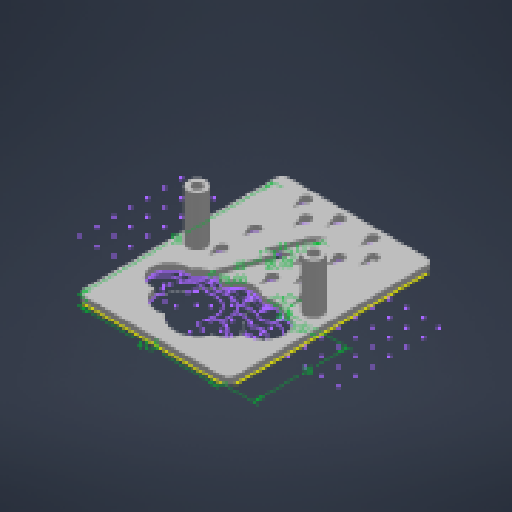
# Autodesk Inventor part: Odbiornik_top
Saved by Autodesk Inventor 2024.4 (Build 284460000, 460)
## iProperties
Created: 2026-02-27
Part Number: Odbiornik_top
Material: Ogólny
Document SubType Name: Modeling
Designer: User
Density: 1 g/cm^3
Appearance: Domyślna
Mass: 5.46546 g
Surface Area: 70.3735 cm^2
Volume: 5.46546 cm^3
Author: User
Autodesk Inventor part; units mm, degrees
ref_plane "YZ Plane" through (0, 0, 0) normal (1, 0, 0) x (0, 1, 0)
ref_plane "XZ Plane" through (0, 0, 0) normal (0, 1, 0) x (-1, 0, 0)
ref_plane "XY Plane" through (0, 0, 0) normal (0, 0, 1) x (1, 0, 0)
sketch "Szkic1" plane through (0, 0, 0) normal (0, 1, 0) x (-1, 0, 0)
  line L0 (-22.5, 30.5) -> (22.5, 30.5)
  line L1 (22.5, 30.5) -> (22.5, -30.5)
  line L2 (22.5, -30.5) -> (-22.5, -30.5)
  line L3 (-22.5, -30.5) -> (-22.5, 30.5)
  line L4 (-22.5, 30.5) -> (22.5, -30.5) construction
  line L5 (22.5, 30.5) -> (16.6, 30.5)
  line L6 (0, -30.5) -> (0, 30.5)
  line L7 (22.5, 0) -> (-22.5, 0)
  line L8 (0, 0) -> (22.5, 0)
  line L9 (22.5, 0) -> (17.38, 0)
  circle A0 centre (17.38, 0) radius 1.5
  circle A1 centre (-17.38, 0) radius 1.5
  circle A2 centre (17.38, 0) radius 2.75
  circle A3 centre (-17.38, 0) radius 2.75
  dimension "d0" = 45
  dimension "d1" = 61
  dimension "d12" = 5.12
  dimension "d13" = 3
  dimension "d14" = 30.5
  dimension "d16" = 5.5
  constraints: 20 end point, 5 midpoint, 4 centre point, 2 coincident, 2 parallel, 2 perpendicular, 2 point on line, 2 symmetric about line, 1 horizontal, 2 other
  measures "d0" distance of L1.end L2.end
  measures "d1" distance of L0.end L1.end
  measures "d12" distance of L7.start L9.end
  measures "d13" diameter of A0
  measures "d14" distance from line of L2 A0.centre
  measures "d16" diameter of A2
extrude "Wyciągnięcie proste1" add sketch "Szkic1" along normal blind 2
extrude "Wyciągnięcie proste2" add sketch "Szkic1" along normal blind 16.8 contours A3 L7 A1 | L7 A1 A3 | A2 L7 A0 | L7 A0 A2
fillet "Zaokrąglenie1" radius 2 4 edges at (-22.5, 1, -30.5) (22.5, 1, -30.5) (-22.5, 1, 30.5) (22.5, 1, 30.5)
sketch "Szkic2" plane through (0, 0, 0) normal (0, -1, 0) x (1, 0, 0)
  line L0 (-21.3296, 27.1767) -> (19.4219, 27.1767) construction
  line L1 (19.4219, 27.1767) -> (19.4219, 1.9055) construction
  line L2 (19.4219, 1.9055) -> (-21.3296, 1.9055) construction
  line L3 (-21.3296, 1.9055) -> (-21.3296, 27.1767) construction
  arc A0 (-12.0648, 18.0488) -> (-11.6976, 7.6041) centre (-12.7532, 12.7958) ccw
  arc A1 (-4.0274, 22.9506) -> (-12.0648, 18.0488) centre (-6.2944, 17.6274) ccw
  arc A2 (8.5818, 21.2572) -> (-4.0274, 22.9506) centre (1.8261, 18.7454) ccw
  arc A3 (12.8836, 16.997) -> (8.5818, 21.2572) centre (7.5717, 15.9353) ccw
  arc A4 (13.1567, 4.5998) -> (12.8836, 16.997) centre (13.0201, 10.7984) ccw
  arc A5 (5.8616, 3.9573) -> (13.1567, 4.5998) centre (8.9779, 10.3115) ccw
  arc A6 (-3.8391, 6.0403) -> (5.8616, 3.9573) centre (1.7998, 8.6711) ccw
  arc A7 (-11.6976, 7.6041) -> (-3.8391, 6.0403) centre (-7.052, 10.4219) ccw
  arc A8 (-4.2074, 7.6238) -> (1.2341, 16.8874) centre (-1.0275, 11.9859) ccw
  arc A9 (-11.7503, 10.9688) -> (-4.2074, 7.6238) centre (-7.2953, 10.8377) ccw
  arc A10 (-17.5377, 13.4696) -> (-11.6516, 9.8959) centre (-12.6699, 14.853) ccw
  arc A11 (3.697, 14.5972) -> (8.6049, 17.9558) centre (3.8701, 19.6096) ccw
  arc A12 (8.6049, 17.9558) -> (11.4505, 18.7493) centre (9.522, 20.1659) ccw
  arc A13 (4.0342, 10.11) -> (9.8976, 11.5253) centre (5.9899, 14.8611) ccw
  arc A14 (9.8976, 11.5253) -> (15.929, 15.2269) centre (12.4747, 14.0908) ccw
  arc A15 (2.5761, 7.9667) -> (9.7755, 8.6284) centre (5.7685, 12.7291) ccw
  arc A16 (9.7755, 8.6284) -> (16.9382, 14.9131) centre (13.3568, 11.7708) ccw
  arc A17 (6.5881, 21.4672) -> (5.2016, 25.1136) centre (2.4919, 21.9965) ccw
  arc A18 (8.5818, 21.2572) -> (6.5881, 21.4672) centre (7.4205, 19.8009) ccw
  arc A19 (10.5725, 13.6586) -> (9.9908, 20.782) centre (6.7774, 16.9342) ccw
  arc A20 (10.5725, 13.6586) -> (12.8792, 16.8923) centre (9.671, 16.7412) ccw
  arc A21 (15.929, 15.2269) -> (15.0518, 16.6562) centre (12.4747, 14.0908) ccw
  arc A22 (16.9382, 14.9131) -> (16.3778, 16.0107) centre (0.1209, 7.0188) ccw
  arc A23 (-11.7503, 10.9688) -> (-5.6989, 9.2808) centre (-8.2416, 11.8564) ccw
  arc A24 (-5.6989, 9.2808) -> (1.2341, 16.8874) centre (-3.3438, 14.0971) ccw
  arc A25 (-11.9834, 18.6814) -> (-11.3996, 15.8747) centre (-9.0372, 17.8302) ccw
  line L4 (-17.5377, 13.4696) -> (-17.7253, 14.625)
  circle A26 centre (12.5, 2.5) radius 1.5
  line L5 (12.5, 2.5) -> (12.5, 6.5)
  arc A27 (12.5, 6.5) -> (13.998, 2.4218) centre (38.5202, 13.7434) ccw
  arc A28 (11.002, 2.4218) -> (12.5, 6.5) centre (-13.5202, 13.7434) ccw
  line L6 (19.4219, 1.9055) -> (19.4219, -1.6866) construction
  line L7 (7.5, 2.5) -> (7.5, 6.5)
  arc A29 (7.5, 6.5) -> (8.998, 2.4218) centre (33.5202, 13.7434) ccw
  circle A30 centre (7.5, 2.5) radius 1.5
  arc A31 (6.002, 2.4218) -> (7.5, 6.5) centre (-18.5202, 13.7434) ccw
  line L8 (2.5, 2.5) -> (2.5, 6.5)
  arc A32 (2.5, 6.5) -> (3.998, 2.4218) centre (28.5202, 13.7434) ccw
  circle A33 centre (2.5, 2.5) radius 1.5
  arc A34 (1.002, 2.4218) -> (2.5, 6.5) centre (-23.5202, 13.7434) ccw
  line L9 (-2.5, 2.5) -> (-2.5, 6.5)
  arc A35 (-2.5, 6.5) -> (-1.002, 2.4218) centre (23.5202, 13.7434) ccw
  circle A36 centre (-2.5, 2.5) radius 1.5
  arc A37 (-3.998, 2.4218) -> (-2.5, 6.5) centre (-28.5202, 13.7434) ccw
  line L10 (-7.5, 2.5) -> (-7.5, 6.5)
  arc A38 (-7.5, 6.5) -> (-6.002, 2.4218) centre (18.5202, 13.7434) ccw
  circle A39 centre (-7.5, 2.5) radius 1.5
  arc A40 (-8.998, 2.4218) -> (-7.5, 6.5) centre (-33.5202, 13.7434) ccw
  line L11 (-12.5, 2.5) -> (-12.5, 6.5)
  arc A41 (-12.5, 6.5) -> (-11.002, 2.4218) centre (13.5202, 13.7434) ccw
  circle A42 centre (-12.5, 2.5) radius 1.5
  arc A43 (-13.998, 2.4218) -> (-12.5, 6.5) centre (-38.5202, 13.7434) ccw
  line L12 (12.5, -2.5) -> (12.5, 1.5)
  arc A44 (12.5, 1.5) -> (13.998, -2.5782) centre (38.5202, 8.7434) ccw
  circle A45 centre (12.5, -2.5) radius 1.5
  arc A46 (11.002, -2.5782) -> (12.5, 1.5) centre (-13.5202, 8.7434) ccw
  line L13 (7.5, -2.5) -> (7.5, 1.5)
  arc A47 (7.5, 1.5) -> (8.998, -2.5782) centre (33.5202, 8.7434) ccw
  circle A48 centre (7.5, -2.5) radius 1.5
  arc A49 (6.002, -2.5782) -> (7.5, 1.5) centre (-18.5202, 8.7434) ccw
  line L14 (2.5, -2.5) -> (2.5, 1.5)
  arc A50 (2.5, 1.5) -> (3.998, -2.5782) centre (28.5202, 8.7434) ccw
  circle A51 centre (2.5, -2.5) radius 1.5
  arc A52 (1.002, -2.5782) -> (2.5, 1.5) centre (-23.5202, 8.7434) ccw
  line L15 (-2.5, -2.5) -> (-2.5, 1.5)
  arc A53 (-2.5, 1.5) -> (-1.002, -2.5782) centre (23.5202, 8.7434) ccw
  circle A54 centre (-2.5, -2.5) radius 1.5
  arc A55 (-3.998, -2.5782) -> (-2.5, 1.5) centre (-28.5202, 8.7434) ccw
  line L16 (-7.5, -2.5) -> (-7.5, 1.5)
  arc A56 (-7.5, 1.5) -> (-6.002, -2.5782) centre (18.5202, 8.7434) ccw
  circle A57 centre (-7.5, -2.5) radius 1.5
  arc A58 (-8.998, -2.5782) -> (-7.5, 1.5) centre (-33.5202, 8.7434) ccw
  line L17 (-12.5, -2.5) -> (-12.5, 1.5)
  arc A59 (-12.5, 1.5) -> (-11.002, -2.5782) centre (13.5202, 8.7434) ccw
  circle A60 centre (-12.5, -2.5) radius 1.5
  arc A61 (-13.998, -2.5782) -> (-12.5, 1.5) centre (-38.5202, 8.7434) ccw
  line L18 (12.5, -7.5) -> (12.5, -3.5)
  arc A62 (12.5, -3.5) -> (13.998, -7.5782) centre (38.5202, 3.7434) ccw
  circle A63 centre (12.5, -7.5) radius 1.5
  arc A64 (11.002, -7.5782) -> (12.5, -3.5) centre (-13.5202, 3.7434) ccw
  line L19 (7.5, -7.5) -> (7.5, -3.5)
  arc A65 (7.5, -3.5) -> (8.998, -7.5782) centre (33.5202, 3.7434) ccw
  circle A66 centre (7.5, -7.5) radius 1.5
  arc A67 (6.002, -7.5782) -> (7.5, -3.5) centre (-18.5202, 3.7434) ccw
  line L20 (2.5, -7.5) -> (2.5, -3.5)
  arc A68 (2.5, -3.5) -> (3.998, -7.5782) centre (28.5202, 3.7434) ccw
  circle A69 centre (2.5, -7.5) radius 1.5
  arc A70 (1.002, -7.5782) -> (2.5, -3.5) centre (-23.5202, 3.7434) ccw
  line L21 (-2.5, -7.5) -> (-2.5, -3.5)
  arc A71 (-2.5, -3.5) -> (-1.002, -7.5782) centre (23.5202, 3.7434) ccw
  circle A72 centre (-2.5, -7.5) radius 1.5
  arc A73 (-3.998, -7.5782) -> (-2.5, -3.5) centre (-28.5202, 3.7434) ccw
  line L22 (-7.5, -7.5) -> (-7.5, -3.5)
  arc A74 (-7.5, -3.5) -> (-6.002, -7.5782) centre (18.5202, 3.7434) ccw
  circle A75 centre (-7.5, -7.5) radius 1.5
  arc A76 (-8.998, -7.5782) -> (-7.5, -3.5) centre (-33.5202, 3.7434) ccw
  line L23 (-12.5, -7.5) -> (-12.5, -3.5)
  arc A77 (-12.5, -3.5) -> (-11.002, -7.5782) centre (13.5202, 3.7434) ccw
  circle A78 centre (-12.5, -7.5) radius 1.5
  arc A79 (-13.998, -7.5782) -> (-12.5, -3.5) centre (-38.5202, 3.7434) ccw
  line L24 (12.5, -12.5) -> (12.5, -8.5)
  arc A80 (12.5, -8.5) -> (13.998, -12.5782) centre (38.5202, -1.2566) ccw
  circle A81 centre (12.5, -12.5) radius 1.5
  arc A82 (11.002, -12.5782) -> (12.5, -8.5) centre (-13.5202, -1.2566) ccw
  line L25 (7.5, -12.5) -> (7.5, -8.5)
  arc A83 (7.5, -8.5) -> (8.998, -12.5782) centre (33.5202, -1.2566) ccw
  circle A84 centre (7.5, -12.5) radius 1.5
  arc A85 (6.002, -12.5782) -> (7.5, -8.5) centre (-18.5202, -1.2566) ccw
  line L26 (2.5, -12.5) -> (2.5, -8.5)
  arc A86 (2.5, -8.5) -> (3.998, -12.5782) centre (28.5202, -1.2566) ccw
  circle A87 centre (2.5, -12.5) radius 1.5
  arc A88 (1.002, -12.5782) -> (2.5, -8.5) centre (-23.5202, -1.2566) ccw
  line L27 (-2.5, -12.5) -> (-2.5, -8.5)
  arc A89 (-2.5, -8.5) -> (-1.002, -12.5782) centre (23.5202, -1.2566) ccw
  circle A90 centre (-2.5, -12.5) radius 1.5
  arc A91 (-3.998, -12.5782) -> (-2.5, -8.5) centre (-28.5202, -1.2566) ccw
  line L28 (-7.5, -12.5) -> (-7.5, -8.5)
  arc A92 (-7.5, -8.5) -> (-6.002, -12.5782) centre (18.5202, -1.2566) ccw
  circle A93 centre (-7.5, -12.5) radius 1.5
  arc A94 (-8.998, -12.5782) -> (-7.5, -8.5) centre (-33.5202, -1.2566) ccw
  line L29 (-12.5, -12.5) -> (-12.5, -8.5)
  arc A95 (-12.5, -8.5) -> (-11.002, -12.5782) centre (13.5202, -1.2566) ccw
  circle A96 centre (-12.5, -12.5) radius 1.5
  arc A97 (-13.998, -12.5782) -> (-12.5, -8.5) centre (-38.5202, -1.2566) ccw
  line L30 (12.5, -17.5) -> (12.5, -13.5)
  arc A98 (12.5, -13.5) -> (13.998, -17.5782) centre (38.5202, -6.2566) ccw
  circle A99 centre (12.5, -17.5) radius 1.5
  arc A100 (11.002, -17.5782) -> (12.5, -13.5) centre (-13.5202, -6.2566) ccw
  line L31 (7.5, -17.5) -> (7.5, -13.5)
  arc A101 (7.5, -13.5) -> (8.998, -17.5782) centre (33.5202, -6.2566) ccw
  circle A102 centre (7.5, -17.5) radius 1.5
  arc A103 (6.002, -17.5782) -> (7.5, -13.5) centre (-18.5202, -6.2566) ccw
  line L32 (2.5, -17.5) -> (2.5, -13.5)
  arc A104 (2.5, -13.5) -> (3.998, -17.5782) centre (28.5202, -6.2566) ccw
  circle A105 centre (2.5, -17.5) radius 1.5
  arc A106 (1.002, -17.5782) -> (2.5, -13.5) centre (-23.5202, -6.2566) ccw
  line L33 (-2.5, -17.5) -> (-2.5, -13.5)
  arc A107 (-2.5, -13.5) -> (-1.002, -17.5782) centre (23.5202, -6.2566) ccw
  circle A108 centre (-2.5, -17.5) radius 1.5
  arc A109 (-3.998, -17.5782) -> (-2.5, -13.5) centre (-28.5202, -6.2566) ccw
  line L34 (-7.5, -17.5) -> (-7.5, -13.5)
  arc A110 (-7.5, -13.5) -> (-6.002, -17.5782) centre (18.5202, -6.2566) ccw
  circle A111 centre (-7.5, -17.5) radius 1.5
  arc A112 (-8.998, -17.5782) -> (-7.5, -13.5) centre (-33.5202, -6.2566) ccw
  line L35 (-12.5, -17.5) -> (-12.5, -13.5)
  arc A113 (-12.5, -13.5) -> (-11.002, -17.5782) centre (13.5202, -6.2566) ccw
  circle A114 centre (-12.5, -17.5) radius 1.5
  arc A115 (-13.998, -17.5782) -> (-12.5, -13.5) centre (-38.5202, -6.2566) ccw
  line L36 (12.5, -22.5) -> (12.5, -18.5)
  arc A116 (12.5, -18.5) -> (13.998, -22.5782) centre (38.5202, -11.2566) ccw
  circle A117 centre (12.5, -22.5) radius 1.5
  arc A118 (11.002, -22.5782) -> (12.5, -18.5) centre (-13.5202, -11.2566) ccw
  line L37 (7.5, -22.5) -> (7.5, -18.5)
  arc A119 (7.5, -18.5) -> (8.998, -22.5782) centre (33.5202, -11.2566) ccw
  circle A120 centre (7.5, -22.5) radius 1.5
  arc A121 (6.002, -22.5782) -> (7.5, -18.5) centre (-18.5202, -11.2566) ccw
  line L38 (2.5, -22.5) -> (2.5, -18.5)
  arc A122 (2.5, -18.5) -> (3.998, -22.5782) centre (28.5202, -11.2566) ccw
  circle A123 centre (2.5, -22.5) radius 1.5
  arc A124 (1.002, -22.5782) -> (2.5, -18.5) centre (-23.5202, -11.2566) ccw
  line L39 (-2.5, -22.5) -> (-2.5, -18.5)
  arc A125 (-2.5, -18.5) -> (-1.002, -22.5782) centre (23.5202, -11.2566) ccw
  circle A126 centre (-2.5, -22.5) radius 1.5
  arc A127 (-3.998, -22.5782) -> (-2.5, -18.5) centre (-28.5202, -11.2566) ccw
  line L40 (-7.5, -22.5) -> (-7.5, -18.5)
  arc A128 (-7.5, -18.5) -> (-6.002, -22.5782) centre (18.5202, -11.2566) ccw
  circle A129 centre (-7.5, -22.5) radius 1.5
  arc A130 (-8.998, -22.5782) -> (-7.5, -18.5) centre (-33.5202, -11.2566) ccw
  line L41 (-12.5, -22.5) -> (-12.5, -18.5)
  arc A131 (-12.5, -18.5) -> (-11.002, -22.5782) centre (13.5202, -11.2566) ccw
  circle A132 centre (-12.5, -22.5) radius 1.5
  arc A133 (-13.998, -22.5782) -> (-12.5, -18.5) centre (-38.5202, -11.2566) ccw
  line L42 (22.5, 28.5) -> (22.5, -28.5) projected
  line L43 (-20.5, 30.5) -> (20.5, 30.5) projected
  line L44 (12.5, -27.5) -> (12.5, -23.5)
  arc A134 (12.5, -23.5) -> (13.998, -27.5782) centre (38.5202, -16.2566) ccw
  circle A135 centre (12.5, -27.5) radius 1.5
  arc A136 (11.002, -27.5782) -> (12.5, -23.5) centre (-13.5202, -16.2566) ccw
  line L45 (7.5, -27.5) -> (7.5, -23.5)
  arc A137 (7.5, -23.5) -> (8.998, -27.5782) centre (33.5202, -16.2566) ccw
  circle A138 centre (7.5, -27.5) radius 1.5
  arc A139 (6.002, -27.5782) -> (7.5, -23.5) centre (-18.5202, -16.2566) ccw
  line L46 (2.5, -27.5) -> (2.5, -23.5)
  arc A140 (2.5, -23.5) -> (3.998, -27.5782) centre (28.5202, -16.2566) ccw
  circle A141 centre (2.5, -27.5) radius 1.5
  arc A142 (1.002, -27.5782) -> (2.5, -23.5) centre (-23.5202, -16.2566) ccw
  line L47 (-2.5, -27.5) -> (-2.5, -23.5)
  arc A143 (-2.5, -23.5) -> (-1.002, -27.5782) centre (23.5202, -16.2566) ccw
  circle A144 centre (-2.5, -27.5) radius 1.5
  arc A145 (-3.998, -27.5782) -> (-2.5, -23.5) centre (-28.5202, -16.2566) ccw
  line L48 (-7.5, -27.5) -> (-7.5, -23.5)
  arc A146 (-7.5, -23.5) -> (-6.002, -27.5782) centre (18.5202, -16.2566) ccw
  circle A147 centre (-7.5, -27.5) radius 1.5
  arc A148 (-8.998, -27.5782) -> (-7.5, -23.5) centre (-33.5202, -16.2566) ccw
  line L49 (-12.5, -27.5) -> (-12.5, -23.5)
  arc A149 (-12.5, -23.5) -> (-11.002, -27.5782) centre (13.5202, -16.2566) ccw
  circle A150 centre (-12.5, -27.5) radius 1.5
  arc A151 (-13.998, -27.5782) -> (-12.5, -23.5) centre (-38.5202, -16.2566) ccw
  line L50 (-8.1124, 5.0931) -> (-2.9821, -9.0023)
  line L51 (-8.1124, 5.0931) -> (6.8876, 5.0931) construction
  line L52 (-2.9821, -9.0023) -> (-5.8799, -8.2259)
  line L53 (-5.8799, -8.2259) -> (-2.1177, -18.5625)
  line L54 (-2.9821, -9.0023) -> (-1.0519, -8.4789)
  line L55 (-1.0519, -8.4789) -> (-5.9916, 5.0931)
  line L56 (-1.0519, -8.4789) -> (-0.0258, -11.298)
  line L57 (-0.0258, -11.298) -> (-2.9236, -10.5215)
  line L58 (-2.9236, -10.5215) -> (0.8386, -20.8581)
  line L59 (-2.1177, -18.5625) -> (0.8386, -20.8581)
  line L60 (20.75, -29) -> (-20.75, -29)
  line L61 (-20.75, -29) -> (-20.75, 29)
  line L62 (-20.75, 29) -> (20.75, 29)
  line L63 (20.75, 29) -> (20.75, -29)
  line L64 (20.75, -29) -> (-20.75, 29) construction
  line L65 (-20.75, -29) -> (20.75, 29) construction
  point P0 (0, 0)
  point P1 (-12.0958, 18.0528)
  point P2 (11.002, 2.4218)
  point P3 (13.4697, -21.3556)
  point P4 (11.5303, -21.3556)
  point P5 (-11.5303, -26.3556)
  point P6 (-13.4697, -26.3556)
  point P7 (-1.5303, -26.3556)
  point P8 (-3.4697, -26.3556)
  point P9 (8.4697, -26.3556)
  point P10 (6.5303, -26.3556)
  point P11 (-6.5303, -21.3556)
  point P12 (-8.4697, -21.3556)
  point P13 (-13.4697, -11.3556)
  point P14 (-11.5303, -11.3556)
  point P15 (3.4697, -1.3556)
  point P16 (1.5303, -1.3556)
  point P17 (11.5303, -1.3556)
  point P18 (13.4697, -1.3556)
  point P19 (6.5303, -6.3556)
  point P20 (8.4697, -6.3556)
  point P21 (3.4697, -11.3556)
  point P22 (1.5303, -11.3556)
  point P23 (8.4697, -16.3556)
  point P24 (6.5303, -16.3556)
  point P25 (-2.6863, -3.9884)
  point P26 (-3.5994, -1.4796)
  point P27 (-7.0312, 4.9886)
  point P28 (-6.5303, 3.6444)
  point P29 (-6.7056, 1.2277)
  point P30 (-7.5, 3.4104)
  point P31 (-7.7093, 3.9853)
  point P32 (-7.5, 4)
  point P33 (-13.4697, -1.3556)
  point P34 (-11.5303, -1.3556)
  dimension "d52" = 3
  dimension "d53" = 4
  dimension "d65" = 5
  dimension "d68" = 5
  dimension "d72" = 10
  dimension "d73" = 28
  dimension "d75" = 15
  dimension "d76" = 70
  dimension "d77" = 3
  dimension "d78" = 55
  dimension "d79" = 11
  dimension "d80" = 2
  dimension "d81" = 3
  dimension "d82" = 3
  dimension "d85" = 11
  dimension "d90" = 41.5
  dimension "d91" = 58
  constraints: 236 point on circle, 120 end point, 110 centre point, 39 vertical, 8 horizontal, 4 parallel, 2 midpoint, 2 point on line, 2 symmetric about line, 1 concentric, 1 equal length, 1 perpendicular, 498 other
  measures "d53" distance of L5.start L5.end
  measures "d65" distance of A28.start A31.start
  measures "d68" distance of A28.start A46.start
  measures "d72" distance from line of L42 L5.start
  measures "d73" distance from line of L43 L5.start
  measures "d75" distance of L50.start L50.end
  measures "d76" angle of L50 L51
  measures "d77" distance of L50.end L52.end
  measures "d78" angle of L50 L52
  measures "d79" distance of L52.end L53.end
  measures "d80" distance of L50.end L54.end
  measures "d81" distance of L54.end L56.end
  measures "d82" distance of L57.start L57.end
  measures "d85" distance of L58.start L58.end
  measures "d90" distance of L61.end L62.end
  measures "d91" distance of L60.end L61.end
extrude "Wyciągnięcie proste9" cut sketch "Szkic2" against normal blind 4.15 contours L4 A10 A9 A40 A7 A0 | A0 A1 A2 A17 A18 A3 A19 A12 A11 A8 A24 A23 A9 A10 L4 | A25 A1 A0 | A9 A23 A24 A8 A38 A40 | A40 A9 L10 A7 | A40 L10 A9 | L10 A9 A38 A7 | A2 A18 A17 | L10 A38 A9 | A38 A9 A8 A15 A16 A22 A4 A5 A27 A28 A30 A29 A31 A6 A33 A32 A34 A36 A35 A37 A7 | A3 A4 A21 A14 A13 A8 A11 A12 A19 | A13 A14 A21 A4 A22 A16 A15 A8 | A37 L9 A6 | L9 A35 A36 A6 | A36 A35 A6 | A36 A6 A35 | A5 L5 A27 | A33 A34 A6 | A5 A26 A28 L5 | A34 A33 A32 A6 | A34 L8 A33 | A5 A26 | A32 A33 A6 | L8 A32 A33 | A5 A29 A30 | A5 L7 A30 A29 | A30 L7 A29 | A5 A30 L7 | L7 A30 A5 A31 picked at (-1.8289, 3.6979) picked at (-1.3724, 3.4401) picked at (1.2391, 3.0886) picked at (3.7517, 3.2083) picked at (8.6294, 3.4279)
extrude "Wyciągnięcie proste10" cut sketch "Szkic2" against normal blind 6.9 contours A150 A151 A149 | A7 A40 L50 | A7 L10 A39 L50 A40 | A7 A38 A39 L10 | A39 L10 L50 | A7 L55 A54 A73 A72 L50 A39 A38 | A39 A38 L50 L10 | A39 A38 | L55 A55 A54 | A72 A73 L50 | A55 L55 A54 | A73 L55 L21 A72 | A72 L55 L54 A89 A91 L50 A73 | L21 L55 A72 | A72 L54 L50 | L54 A91 A72 | A72 A91 A90 A109 L53 L52 L54 | L55 L54 A72 | A91 L54 L27 A72 | A72 L27 L57 L58 A90 A91 | A91 L27 L54 | L54 L56 L57 A89 A72 | A72 A89 L54 | L27 L54 A89 A72 | A72 A89 L57 L27 | A91 A90 | A90 L58 A107 A109 A91 | A89 L54 L27 | A109 A90 L33 A108 L53 | A109 L33 A90 | A108 A107 L59 L53 | A52 L14 A33 | A33 L14 A51 A52 | L33 A107 A90 | A90 A107 A108 L33 | A44 A45 L12 A26 | A26 L12 A44 | L14 A50 A33 | A33 A50 A51 L14 | A52 A51 | A51 A50 A68 A70 A52 | L58 L59 A108 A107 A90 | A108 A107 | L12 A45 A46 A26 | A26 A46 L12 | A45 A44 | A44 A45 A62 A64 A46 | A51 A50 | A70 L20 A51 | A46 A45 | A45 L18 A62 | L20 A68 A51 | A130 L40 A111 | A111 L40 A129 A130 | A145 L47 A126 | A126 L47 A144 A145 | A45 A64 L18 | L40 A128 A111 | A111 A128 A129 L40 | A130 A129 | A129 A128 A146 A148 A130 | L47 A143 A126 | A126 A143 A144 L47 | A145 A144 | A144 A143 A145 | A88 L26 A69 | A69 L26 A87 A88 | A129 A128 | A144 A143 | A65 A66 L19 A48 | A48 L19 A65 | L26 A86 A69 | A69 A86 A87 L26 | A88 A87 | A87 A86 A104 A106 A88 | A148 L48 A129 | L19 A66 A67 A48 | A48 A67 L19 | A66 A65 | A65 A66 A83 A85 A67 | L48 A146 A129 | A87 A86 | A106 L32 A87 | A138 A139 A137 | A67 A66 | A66 L25 A83 | L32 A104 A87 | A138 A139 | A137 A138 | A150 A151 | A149 A150 | A66 A85 L25 | A139 A120 L45 A138 | A138 L45 A120 A137 | A151 A132 L49 A150 | A150 L49 A132 A149 | A139 L45 A120 | A120 L45 A137 | A151 L49 A132 | A132 L49 A149 | A101 A102 L31 A84 | A84 L31 A101 | A116 A117 L36 A99 | A99 L36 A116 | A136 L44 A117 | A117 A118 A116 A134 A136 | A117 L44 A134 | L31 A102 A103 A84 | A84 A103 L31 | A102 A101 | A101 A102 A119 A121 A103 | L36 A117 A118 A99 | A99 A118 L36 | A117 A116 | A117 A118 | A121 L37 A102 | A102 L37 A119 | A103 A102 | A115 L35 A96 | A96 A97 A95 A113 A115 | A96 L35 A113 | A96 A97 | A95 A96 | A97 A78 L29 A96 | A96 L29 A78 A95 | A97 L29 A78 | A78 L29 A95 | A79 L23 A60 | A60 A61 A59 A77 A79 | A60 L23 A77 | A60 A61 | A59 A60 | A61 A42 L17 A60 | A60 L17 A42 A59 | A61 L17 A42 | A42 L17 A59 picked at (-3.8204, -2.0508) picked at (-3.7207, -6.8265) picked at (-3.4125, -2.7175)
